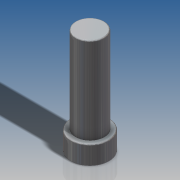
# Autodesk Inventor part: u9208
Saved by Autodesk Inventor 2016 SP2 (Build 200236200, 236)
## iProperties
Created: 2015-08-21
Part Number: u9208
Material: Steel
Document SubType Name: Modeling
Designer: D. Kohfeld
Mass: 0.356245 g
Surface Area: 0.852567 cm^2
Volume: 0.0453816 cm^3
Density: 7.85 g/cm^3
Appearance: ElectricAlloy
Author: D. Kohfeld
Autodesk Inventor part; units mm, degrees
ref_plane "YZ Plane" through (0, 0, 0) normal (1, 0, 0) x (0, 1, 0)
ref_plane "XZ Plane" through (0, 0, 0) normal (0, 1, 0) x (-1, 0, 0)
ref_plane "XY Plane" through (0, 0, 0) normal (0, 0, 1) x (1, 0, 0)
sketch "Sketch2" plane through (0, 0, 0) normal (0, 0, 1) x (1, 0, 0)
  line L0 (1.2, 0) -> (1.6, 0)
  line L1 (1.6, 0) -> (1.6, -1.6)
  line L2 (1.6, -1.6) -> (0, -1.6)
  line L3 (0, -1.6) -> (0, 7.2)
  line L4 (0, 7.2) -> (1.2, 7.2)
  line L5 (1.2, 7.2) -> (1.2, 0)
  point P0 (0, 0)
  dimension "d0" = 3.2
  dimension "d1" = 2.4
  dimension "d2" = 1.6
  dimension "d3" = 7.2
  constraints: 12 end point, 3 horizontal, 3 vertical, 1 horizontal alignment, 1 point on line
  measures "d0" diameter of L1 L3
  measures "d1" diameter of L5 L3
  measures "d2" distance of L0.end L1.end
  measures "d3" distance of L4.end L0.start
revolve "Revolution1" add sketch "Sketch2" angle 360 about axis through (0, -1.6, 0) along (0, 1, 0)
fillet "Fillet1" radius 0.1 3 edges at (-1.2, 7.2, 0) (-1.6, 0, 0) (-1.6, -1.6, 0)
body "Solid1"
